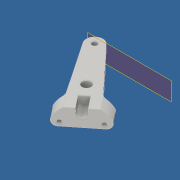
# Autodesk Inventor part: Mount_B
Saved by Autodesk Inventor 2016 (Build 200138000, 138)
## iProperties
Created: 2016-03-27
Part Number: Mount_B
Material: ABS-Kunststoff
Document SubType Name: Modeling
Designer: 4ndreas
Density: 1.06 g/cm^3
Appearance: Glatt - weiß
Mass: 10.4353 g
Surface Area: 46.3478 cm^2
Volume: 9.84464 cm^3
Author: 4ndreas
Autodesk Inventor part; units mm, degrees
ref_plane "YZ Plane" through (0, 0, 0) normal (1, 0, 0) x (0, 1, 0)
ref_plane "XY Plane" through (0, 0, 0) normal (0, 0, 1) x (1, 0, 0)
sketch "Skizze1" plane through (0, 0, 0) normal (0, 0, 1) x (1, 0, 0)
  line L0 (23.3115, -64.9198) -> (53.8426, -40.6536) projected
  circle A0 centre (0, -4.25) radius 6.5
  line L1 (43.6656, -48.7423) -> (33.4885, -56.8311)
  line L2 (33.4885, -56.8311) -> (-5.0885, -8.2944)
  line L3 (-5.0885, -8.2944) -> (5.0885, -0.2056)
  line L4 (5.0885, -0.2056) -> (43.6656, -48.7423)
  point P0 (0, 0)
  dimension "d0" = 13
  constraints: 8 end point, 2 coincident, 2 parallel, 2 point on line, 1 centre point, 1 midpoint, 1 perpendicular, 1 tangent, 1 other
  measures "d0" diameter of A0
extrude "Extrusion1" add sketch "Skizze1" along normal blind 3
sketch "Skizze2" plane through (43.6656, -48.7423, 0) normal (0.6222102, -0.7828502, 0) x (0.7828502, 0.6222102, 0)
  circle A0 centre (-17.7583, -20) radius 1.5 projected
  circle A1 centre (4.7583, -20) radius 1.5 projected
  circle A2 centre (-6.5, -0.5) radius 1.5 projected
  line L0 (-23, -30.5) -> (10, -30.5) projected
  line L1 (10, -30.5) -> (10, -26.4615) projected
  arc A3 (11.0169, -22.0678) -> (10, -26.4615) centre (20, -26.4615) ccw projected
  arc A4 (11.0169, -22.0678) -> (-24.0169, -22.0678) centre (-6.5, -13.5) ccw projected
  arc A5 (-23, -26.4615) -> (-24.0169, -22.0678) centre (-33, -26.4615) ccw projected
  line L2 (-23, -26.4615) -> (-23, -30.5) projected
  line L3 (12.6833, -10) -> (-25.6833, -10)
  line L4 (-104.8912, -12) -> (94.8547, -12)
  line L5 (-13, 3) -> (0, 3) projected
  line L6 (3.8923, 3) -> (-16.8923, 3)
  line L7 (-21.75, -5.4123) -> (-19, -3.8246) projected
  line L8 (-19, -3.8246) -> (-16.25, -5.4123) projected
  line L9 (-16.25, -5.4123) -> (-16.25, -8.5877) projected
  line L10 (-16.25, -8.5877) -> (-19, -10.1754) projected
  line L11 (-19, -10.1754) -> (-21.75, -8.5877) projected
  line L12 (-21.75, -8.5877) -> (-21.75, -5.4123) projected
  line L13 (3.25, -5.4123) -> (6, -3.8246) projected
  line L14 (6, -3.8246) -> (8.75, -5.4123) projected
  line L15 (8.75, -5.4123) -> (8.75, -8.5877) projected
  line L16 (8.75, -8.5877) -> (6, -10.1754) projected
  line L17 (6, -10.1754) -> (3.25, -8.5877) projected
  line L18 (3.25, -8.5877) -> (3.25, -5.4123) projected
  circle A6 centre (-6.5, -13.5) radius 5 projected
  point P0 (-3.8556, 0)
  dimension "d3" = 2
  constraints: 6 end point, 4 point on circle, 2 horizontal, 1 collinear, 2 other
  measures "d3" distance between parallel lines of L4 L3
extrude "Extrusion2" add sketch "Skizze2" against normal blind 12 contours A4 L6 L5 L3 L16 L15 L14 L13 L18 L17 A6 L10 L9 L8 L7 L12 L11 | L11 L12 L7 L8 L9 L10 L3 | A6 L3 | L3 L17 L18 L13 L14 L15 L16
sketch "Skizze3" plane through (0, 0, 3) normal (0, 0, 1) x (1, 0, 0)
  line L0 (36.199, -39.3481) -> (5.0885, -0.2056) projected
  arc A0 (5.0885, -0.2056) -> (-5.0885, -8.2944) centre (0, -4.25) ccw projected
  line L1 (-5.0885, -8.2944) -> (26.022, -47.4369) projected
  line L2 (22.9749, -49.8587) -> (26.022, -47.4369) projected
  line L3 (30.4414, -59.2529) -> (22.9749, -49.8587) projected
  line L4 (46.7127, -46.3205) -> (30.4414, -59.2529) projected
  line L5 (46.7127, -46.3205) -> (39.2461, -36.9263) projected
  line L6 (36.199, -39.3481) -> (39.2461, -36.9263) projected
  line L7 (22.9749, -49.8587) -> (-5.0885, -8.2944)
  line L8 (39.2461, -36.9263) -> (5.0885, -0.2056)
  point P0 (0, 0)
  constraints: 4 end point
extrude "Extrusion3" add sketch "Skizze3" against normal up to surface (3 mm away) contours L0 L8 L6 | L1 L2 L7
sketch "Skizze4" plane through (23.5594, -64.7228, -10) normal (0.6222102, -0.7828502, 0) x (0.7828502, 0.6222102, 0)
  line L0 (29.5756, 13) -> (8.791, 13) projected
  arc A0 (8.791, 13) -> (0, 0) centre (19.1833, -3.5) ccw projected
  line L1 (0, 0) -> (38.3667, 0) projected
  arc A1 (38.3667, 0) -> (29.5756, 13) centre (19.1833, -3.5) ccw projected
  arc A2 (17.7691, 10) -> (20.5975, 10) centre (19.1833, 9.5) ccw projected
  line L2 (17.7691, 10) -> (20.5975, 10) projected
  circle A3 centre (19.1833, 9.5) radius 1.5
  circle A4 centre (19.1833, 9.5) radius 3.5
  point P0 (21.8277, 10)
  dimension "d8" = 7
  constraints: 2 centre point, 2 coincident, 1 concentric
  measures "d8" diameter of A4
extrude "Extrusion4" cut sketch "Skizze4" against normal blind 12 contours A4 | L2 A2 | A3 L2
sketch "Skizze6" plane through (23.5594, -64.7228, -10) normal (0.6222102, -0.7828502, 0) x (0.7828502, 0.6222102, 0)
  circle A0 centre (19.1833, 9.5) radius 3.5 projected
  line L0 (29.5756, 13) -> (19.1833, 13) construction
  arc A1 (8.791, 13) -> (0, 0) centre (19.1833, -3.5) ccw construction
  line L1 (0, 0) -> (38.3667, 0) construction
  arc A2 (38.3667, 0) -> (29.5756, 13) centre (19.1833, -3.5) ccw construction
  line L2 (15.6833, 13) -> (22.6833, 13)
  line L3 (22.6833, 13) -> (22.6833, 9.5)
  line L4 (22.6833, 9.5) -> (15.6833, 9.5)
  line L5 (15.6833, 9.5) -> (15.6833, 13)
  circle A3 centre (19.1833, 9.5) radius 3.5 projected
  line L6 (19.1833, 13) -> (8.791, 13) projected
  point P0 (21.8277, 10)
  point P1 (21.0706, 13)
  point P2 (17.4651, 13)
  constraints: 8 end point, 2 parallel, 1 horizontal, 1 perpendicular, 1 point on circle, 1 point on line, 1 tangent, 2 other
extrude "Extrusion6" cut sketch "Skizze6" against normal up to surface (12 mm away) contours L4 A0 | A0 L2 L3 | A0 L5 L2 picked at (20.0662, 10.487)
sketch "Skizze7" plane through (36.199, -39.3481, 0) normal (-0.6222102, 0.7828502, 0) x (0.7828502, 0.6222102, 0)
  line L0 (-16.8923, -3) -> (-16.8923, 0) projected
  line L1 (-16.8923, 0) -> (-10, 0) projected
  line L2 (3.8923, 0) -> (3.8923, -3) projected
  arc A0 (3.8923, -3) -> (12.6833, 10) centre (-6.5, 13.5) ccw projected
  line L3 (12.6833, 10) -> (-25.6833, 10) projected
  arc A1 (-25.6833, 10) -> (-16.8923, -3) centre (-6.5, 13.5) ccw projected
  circle A2 centre (-19, 7) radius 1.5 projected
  circle A3 centre (6, 7) radius 1.5 projected
  line L4 (-3, 0.5) -> (-3, 0) projected
  line L5 (3.8923, 0) -> (-3, 0) projected
  line L6 (-10, 0) -> (-10, 0.5) projected
  arc A4 (-3, 0.5) -> (-10, 0.5) centre (-6.5, 0.5) ccw projected
  point P0 (-3.8556, 0)
extrude "Extrusion7" cut sketch "Skizze7" against normal through all contours A2 | A3
sketch "Skizze8" plane through (0, 0, 0) normal (0, 0, -1) x (-1, 0, 0)
  line L0 (-22.9749, -49.8587) -> (-28.3705, -45.5702) projected
  line L1 (-22.9749, -49.8587) -> (5.0885, -8.2944) projected
  arc A0 (5.0885, -8.2944) -> (-5.0885, -0.2056) centre (0, -4.25) ccw projected
  line L2 (-5.0885, -0.2056) -> (-39.2461, -36.9263) projected
  circle A1 centre (0, -4.25) radius 3.5
  line L3 (-33.8505, -41.2148) -> (-28.3705, -45.5702) projected
  line L4 (-39.2461, -36.9263) -> (-33.8505, -41.2148) projected
  point P0 (0, 0)
  dimension "d17" = 7
  constraints: 1 centre point, 1 coincident
  measures "d17" diameter of A1
extrude "Extrusion8" add sketch "Skizze8" along normal blind 0.5 contours A1
chamfer "Fase1" distance 0.5 angle 45 1 edges at (3.5, -4.25, 0)
sketch "Skizze9" plane through (0, 0, 3) normal (0, 0, 1) x (1, 0, 0)
  circle A0 centre (0, -4.25) radius 3.5 projected
  point P0 (0, 0)
hole "Bohrung1" at (0, -4.25, 3) direction (0, 0, -1) diameter 4 end through all
sketch "Skizze10" plane through (0, 0, 3) normal (0, 0, 1) x (1, 0, 0)
  circle A0 centre (24.2662, -34.7812) radius 3.5
  point P0 (0, 0)
  dimension "d30" = 7
  constraints: 1 centre point, 1 coincident, 1 other
  measures "d30" diameter of A0
extrude "Extrusion9" cut sketch "Skizze10" against normal through all
sketch "Skizze11" plane through (0, 0, 0) normal (0, 0, -1) x (-1, 0, 0)
  circle A0 centre (-24.2662, -34.7812) radius 3.5 projected
  line L0 (-22.9749, -49.8587) -> (-28.3705, -45.5702) projected
  line L1 (-22.9749, -49.8587) -> (5.0885, -8.2944) projected
  arc A1 (5.0885, -8.2944) -> (-5.0885, -0.2056) centre (0, -4.25) ccw projected
  line L2 (-5.0885, -0.2056) -> (-39.2461, -36.9263) projected
  circle A2 centre (0, -4.25) radius 4 projected
  arc A3 (-12.4206, -8.0879) -> (-0.9354, -17.2163) centre (0, -4.25) ccw
  line L3 (-22.9749, -49.8587) -> (5.0885, -8.2944) projected
  line L4 (-33.8505, -41.2148) -> (-28.3705, -45.5702) projected
  line L5 (-39.2461, -36.9263) -> (-33.8505, -41.2148) projected
  point P0 (0, 0)
  dimension "d33" = 13
  constraints: 2 point on circle, 2 point on line, 1 centre point, 1 coincident
  measures "d33" radius of A3
extrude "Extrusion10" add sketch "Skizze11" along normal blind 5 contours L0 L4 L5 L2 A3 L1
fillet "Rundung1" radius 2 2 edges at (0.9354, -17.2163, -2.5) (12.4206, -8.0879, -2.5)
fillet "Rundung2" radius 2 8 edges at (2.4138, -17.9483, -5) (8.0887, -14.4271, -5) (12.8, -9.6934, -5) (26.8705, -23.6221, -5) (12.8073, -34.7996, -5) (22.9749, -49.8587, -1) (39.2461, -36.9263, -1) (31.1105, -43.3925, -5)
fillet "Rundung2" radius 4 2 edges at (49.8614, -36.1536, -10) (19.8261, -60.0257, -10)
